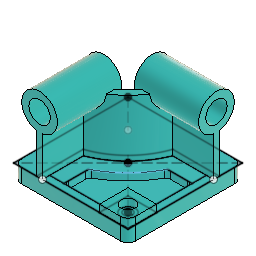
Design 9 v1 (Autodesk Fusion 360 design; units mm, degrees)
Autodesk Fusion 360 part; units mm, degrees
note: some values were not read from the file. Set by a fixed rule: which sketch regions a step uses.
sketch "Sketch1" plane through (0, 0, 0) normal (0, 0, 1) x (1, 0, 0)
  line L0 (200, 200) -> (-200, 200)
  line L1 (-200, 200) -> (-200, -200)
  line L2 (-200, -200) -> (200, -200)
  line L3 (200, -200) -> (200, 200)
  line L4 (200, 200) -> (-200, -200) construction
  line L5 (200, -200) -> (100, -200)
  line L6 (100, -200) -> (100, -100)
  line L7 (100, -100) -> (200, -100)
  line L8 (200, -100) -> (200, -200)
  line L9 (-120, -200) -> (-120, -36.8544)
  line L10 (36.8544, 120) -> (200, 120)
  line L11 (-100, -200) -> (-100, -56.1738)
  line L12 (56.1738, 100) -> (200, 100)
  line L13 (-200, 200) -> (-100, 100) construction
  line L14 (-23.2233, 23.2233) -> (200, -200) construction
  arc A0 (-120, -36.8544) -> (36.8544, 120) centre (-200, 200) ccw
  arc A1 (-100, -56.1738) -> (56.1738, 100) centre (-200, 200) ccw
  line L15 (175, 100) -> (175, -100)
  line L16 (100, -175) -> (-100, -175)
  line L17 (-50, -175) -> (-50, -88.3141)
  arc A2 (-50, -88.3141) -> (88.3141, 50) centre (-200, 200) ccw
  line L18 (88.3141, 50) -> (175, 50)
  circle A3 centre (150, -150) radius 25
  circle A4 centre (150, -150) radius 15
  dimension "d1" = 400
  dimension "d2" = 400
  dimension "d3" = 100
  dimension "d4" = 100
  dimension "d5" = 500
  dimension "d6" = 550
  dimension "d7" = 80
  dimension "d8" = 80
  dimension "d10" = 25
  dimension "d11" = 25
  dimension "d13" = 50
  dimension "d14" = 30
  dimension "d15" = 50
  constraint horizontal L0
  constraint perpendicular L0 L1
  constraint parallel L0 L2
  constraint parallel L1 L3
  constraint coincident L4 origin
  constraint coincident origin L13
  constraint horizontal L5
  constraint vertical L6
  constraint horizontal L7
  constraint vertical L8
  constraint coincident L0.end L1.start
  constraint concentric A0 A1
  constraint coincident L2 L9.start
  constraint perpendicular L2 L9
  constraint coincident L3 L10.end
  constraint perpendicular L3 L10
  constraint coincident L14.start A0
  constraint collinear L13 L14
  constraint coincident L12 L15.start
  constraint coincident L7 L15.end
  constraint perpendicular L7 L15
  constraint coincident L6 L16.start
  constraint coincident L11 L16.end
  constraint perpendicular L11 L16
  constraint concentric A1 A2
  constraint coincident L16 L17.start
  constraint coincident L15 L18.end
  constraint coincident L14 A3.centre
  constraint concentric A3 A4
  measures "d1" distance of L1.end L2.end
  measures "d2" distance of L0.end L1.end
  measures "d3" distance of L2.end L5.end
  measures "d4" distance of L2.end L7.end
  measures "d5" diameter of A0
  measures "d6" diameter of A1
  measures "d7" distance of L0 L10
  measures "d8" distance of L1 L9
  measures "d10" distance of L3 L15
  measures "d11" distance of L2 L16
  measures "d13" diameter of A3
  measures "d14" diameter of A4
  measures "d15" distance of L6 A3.centre
extrude "Extrude1" add sketch "Sketch1" against normal blind 50 contours L0 L1 L2 L3 L9 L10 A0 | L2 L3 L9 L10 L11 L12 A0 A1 | L3 L7 L12 L15 | L2 L3 L5 L6 L7 L8 | L11 L12 A1 L15 L16 L17 A2 L18 | L2 L6 L11 L16 | L6 L7 L15 L16 L17 A2 L18 | A3 | A4
extrude "Extrude2" cut sketch "Sketch1" against normal blind 25 contours L6 L7 L15 L16 L17 A2 L18
extrude "Extrude3" cut sketch "Sketch1" against normal blind 110 contours A4
extrude "Extrude4" add sketch "Sketch1" along normal blind 25 contours L2 L3 L5 L6 L7 L8
extrude "Extrude5" add sketch "Sketch1" along normal blind 200 contours L2 L3 L9 L10 L11 L12 A0 A1
fillet "Fillet1" radius 25 4 edges at (-200, 200, -25) (200, 200, -25) (-200, -200, -25) (200, -200, -12.5)
fillet "Fillet2" radius 15 5 edges at (88.3141, 50, -12.5) (-50, -88.3141, -12.5) (-50, -175, -12.5) (100, -175, -12.5) (175, 50, -12.5)
sketch "Sketch2" plane through (0, -200, 0) normal (0, -1, 0) x (1, 0, 0)
  line L0 (175, -50) -> (175, 25)
  line L1 (175, 25) -> (100, 25)
  line L2 (100, 25) -> (100, 0)
  line L3 (100, 0) -> (-100, 0)
  line L4 (-100, 0) -> (-100, 200)
  line L5 (-100, 200) -> (-120, 200)
  line L6 (-120, 200) -> (-120, 0)
  line L7 (-120, 0) -> (-175, 0)
  line L8 (-175, 0) -> (-175, -50)
  line L9 (-175, -50) -> (175, -50)
  circle A0 centre (-110, 200) radius 62.5
  dimension "d30" = 125
  constraint midpoint L5 A0.centre
  measures "d30" diameter of A0
extrude "Extrude6" add sketch "Sketch2" against normal blind 225 contours L4 L5 L6 A0 | L4 L5 L6 A0
sketch "Sketch3" plane through (200, 0, 0) normal (1, 0, 0) x (0, 1, 0)
  line L0 (-175, 25) -> (-175, -50)
  line L1 (-175, -50) -> (175, -50)
  line L2 (175, -50) -> (175, 0)
  line L3 (175, 0) -> (120, 0)
  line L4 (120, 0) -> (120, 200)
  line L5 (120, 200) -> (100, 200)
  line L6 (100, 200) -> (100, 0)
  line L7 (100, 0) -> (-100, 0)
  line L8 (-100, 0) -> (-100, 25)
  line L9 (-100, 25) -> (-175, 25)
  circle A0 centre (110, 200) radius 62.5
  dimension "d33" = 125
  constraint midpoint L5 A0.centre
  measures "d33" diameter of A0
extrude "Extrude7" add sketch "Sketch3" against normal blind 225 contours L4 L5 L6 A0 | L4 L5 L6 A0
hole "Hole1" at (-110, -200, 200) direction (0, 1, 0) diameter 75 end through all
hole "Hole2" at (200, 110, 200) direction (-1, 0, 0) diameter 75 end through all
